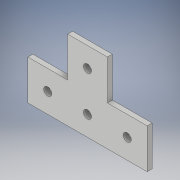
# Autodesk Inventor part: Short T-Gusset
Saved by Autodesk Inventor 2018 (Build 220112000, 112)
## iProperties
Created: 2019-01-19
Part Number: Short T-Gusset
Material: Generic
Document SubType Name: Modeling
Designer: maste
Density: 1 g/cm^3
Appearance: Default
Author: maste
Autodesk Inventor part; units mm, degrees
ref_plane "YZ Plane" through (0, 0, 0) normal (1, 0, 0) x (0, 1, 0)
ref_plane "XZ Plane" through (0, 0, 0) normal (0, 1, 0) x (-1, 0, 0)
ref_plane "XY Plane" through (0, 0, 0) normal (0, 0, 1) x (1, 0, 0)
sketch "Sketch1" plane through (0, 0, 0) normal (0, 0, 1) x (1, 0, 0)
  line L0 (0, 0) -> (0, 25.4)
  line L1 (0, 25.4) -> (25.4, 25.4)
  line L2 (25.4, 25.4) -> (25.4, 50.8)
  line L3 (25.4, 50.8) -> (50.8, 50.8)
  line L4 (50.8, 50.8) -> (50.8, 25.4)
  line L5 (50.8, 25.4) -> (76.2, 25.4)
  line L6 (76.2, 25.4) -> (76.2, 0)
  line L7 (76.2, 0) -> (0, 0)
  line L8 (0, 12.7) -> (12.7, 12.7) construction
  line L9 (12.7, 12.7) -> (38.1, 12.7) construction
  line L10 (38.1, 12.7) -> (63.5, 12.7) construction
  line L11 (38.1, 12.7) -> (38.1, 38.1) construction
  circle A0 centre (38.1, 12.7) radius 2.5797
  circle A1 centre (63.5, 12.7) radius 2.5797
  circle A2 centre (12.7, 12.7) radius 2.5797
  circle A3 centre (38.1, 38.1) radius 2.5797
  dimension "d0" = 25.4
  dimension "d1" = 25.4
  dimension "d2" = 25.4
  dimension "d3" = 25.4
  dimension "d4" = 25.4
  dimension "d5" = 25.4
  dimension "d6" = 12.7
  dimension "d7" = 25.4
  dimension "d8" = 25.4
  dimension "d9" = 5.1594
  constraints: 24 end point, 5 perpendicular, 4 centre point, 4 coincident, 4 point on line, 2 vertical, 1 horizontal, 1 midpoint
  measures "d0" distance of L0.start L0.end
  measures "d1" distance of L0.end L1.end
  measures "d2" distance of L1.end L2.end
  measures "d3" distance of L2.end L3.end
  measures "d4" distance of L3.end L4.end
  measures "d5" distance of L4.end L5.end
  measures "d6" distance of L8.start L8.end
  measures "d7" distance of L8.end L9.end
  measures "d8" distance of L9.end L10.end
  measures "d9" diameter of A0
extrude "Extrusion1" add sketch "Sketch1" along normal blind 3.175
body "Solid1"
